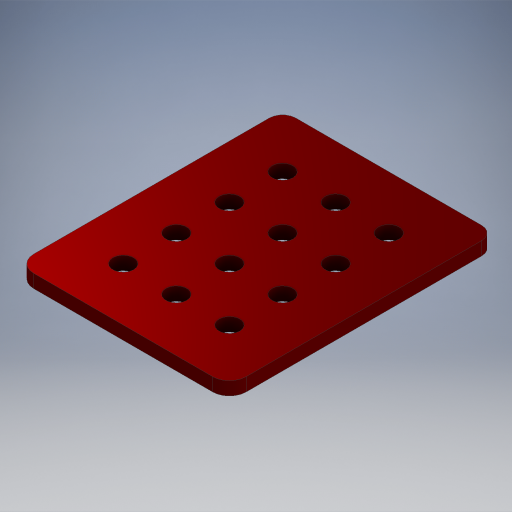
# Autodesk Inventor part: 3x5-Grid-Gusset
Saved by Autodesk Inventor 2024.2 (Build 282272000, 272)
## iProperties
Created: 2024-02-11
Part Number: 3x5-Grid-Gusset
Material: Generic
Document SubType Name: Modeling
Designer: rohan
Density: 1 g/cm^3
Appearance: Default
Author: rohan
Autodesk Inventor part; units mm, degrees
ref_plane "YZ Plane" through (0, 0, 0) normal (1, 0, 0) x (0, 1, 0)
ref_plane "XZ Plane" through (0, 0, 0) normal (0, 1, 0) x (-1, 0, 0)
ref_plane "XY Plane" through (0, 0, 0) normal (0, 0, 1) x (1, 0, 0)
sketch "Sketch1" plane through (0, 0, 0) normal (0, 1, 0) x (-1, 0, 0)
  circle A0 centre (13.0821, 0) radius 2.4892
  circle A1 centre (0.3821, 0) radius 2.4892
  line L0 (0, 10.7252) -> (0, 9.1262) construction
  circle A2 centre (-12.3179, 0) radius 2.4892
  line L1 (21.7943, 12.7) -> (-21.0301, 12.7)
  line L2 (-25.0179, 8.7122) -> (-25.0179, -47.625)
  line L3 (25.7821, -47.625) -> (25.7821, 8.7122)
  arc A3 (25.7821, 8.7122) -> (21.7943, 12.7) centre (21.7943, 8.7122) ccw
  arc A4 (-21.0301, 12.7) -> (-25.0179, 8.7122) centre (-21.0301, 8.7122) ccw
  line L4 (22.6071, -50.8) -> (-21.8429, -50.8)
  arc A5 (22.6071, -50.8) -> (25.7821, -47.625) centre (22.6071, -47.625) ccw
  arc A6 (-25.0179, -47.625) -> (-21.8429, -50.8) centre (-21.8429, -47.625) ccw
  circle A7 centre (13.0821, -12.7) radius 2.4892
  circle A8 centre (0.3821, -12.7) radius 2.4892
  circle A9 centre (-12.3179, -12.7) radius 2.4892
  circle A10 centre (13.0821, -25.4) radius 2.4892
  circle A11 centre (0.3821, -25.4) radius 2.4892
  circle A12 centre (-12.3179, -25.4) radius 2.4892
  circle A13 centre (13.0821, -38.1) radius 2.4892
  circle A14 centre (0.3821, -38.1) radius 2.4892
  circle A15 centre (-12.3179, -38.1) radius 2.4892
  point P0 (0, 0)
  point P1 (-25.0179, 12.7)
  point P2 (25.7821, -50.8)
  dimension "d0" = 4.9784
  dimension "d1" = 4.9784
  dimension "d2" = 12.7
  dimension "d3" = 4.9784
  dimension "d4" = 12.7
  dimension "d16" = 3.9878
  dimension "d20" = 3.175
  dimension "d21" = 50.8
  dimension "d22" = 63.5
  dimension "d25" = 12.7
  constraints: 16 centre point, 10 end point, 8 point on circle, 8 tangent, 4 point on line, 2 equal radius, 2 perpendicular, 2 vertical, 1 horizontal, 1 parallel, 18 other
  measures "d0" diameter of A0
  measures "d1" diameter of A1
  measures "d2" distance of A1.centre A0.centre
  measures "d3" diameter of A2
  measures "d4" distance of A1.centre A2.centre
  measures "d16" radius of A3
  measures "d20" radius of A5
  measures "d21" distance between parallel lines of L2 L3
  measures "d22" distance between parallel lines of L1 L4
  measures "d25" distance of A0.centre A7.centre
extrude "Extrusion1" add sketch "Sketch1" along normal blind 3.175
body "Solid1"
